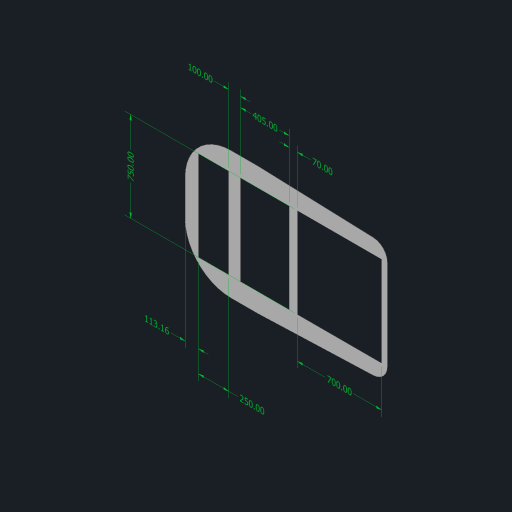
# Autodesk Inventor part: CHAPA_6
Saved by Autodesk Inventor 2024.3 (Build 283343000, 343)
## iProperties
Created: 2024-06-30
Part Number: CHAPA_6
Material: Generic
Document SubType Name: Sheet Metal
Designer: Niler
Density: 1 g/cm^3
Sheet Metal Rule: Default_mm
Appearance: Default
Author: Niler
Autodesk Inventor part; units mm, degrees
ref_plane "YZ Plane" through (0, 0, 0) normal (1, 0, 0) x (0, 1, 0)
ref_plane "XZ Plane" through (0, 0, 0) normal (0, 1, 0) x (-1, 0, 0)
ref_plane "XY Plane" through (0, 0, 0) normal (0, 0, 1) x (1, 0, 0)
sketch "Sketch1" plane through (0, 0, 0) normal (0, 0, 1) x (1, 0, 0)
  arc A0 (216.4448, 899.4448) -> (-166.5552, 516.4448) centre (216.4448, 516.4448) ccw
  line L0 (-166.5552, 216.4448) -> (-166.5552, 516.4448)
  arc A1 (-166.5552, 216.4448) -> (216.4448, -166.5552) centre (216.4448, 216.4448) ccw
  line L1 (443.4448, -166.5552) -> (216.4448, -166.5552)
  line L2 (216.4448, 899.4448) -> (443.4448, 899.4448)
  line L3 (443.5712, 899.4425) -> (1403.908, 864.732)
  line L4 (1403.908, -131.8425) -> (443.5712, -166.5529)
  arc A2 (443.4448, -166.5552) -> (443.5712, -166.5529) centre (443.4448, -163.0552) ccw
  arc A3 (443.5712, 899.4425) -> (443.4448, 899.4448) centre (443.4448, 895.9448) ccw
  arc A4 (1521.5977, 742.7757) -> (1403.908, 864.732) centre (1399.4977, 742.7117) ccw
  line L5 (1521.5977, 742.7757) -> (1521.6067, 725.4805)
  line L6 (1521.6067, 7.4091) -> (1521.5977, -9.8861)
  arc A5 (1403.908, -131.8425) -> (1521.5977, -9.8861) centre (1399.4977, -9.8222) ccw
  line L7 (1521.6067, 725.4805) -> (1521.6067, 7.4091)
  point P0 (0, 0)
extrude "Plate1" add sketch "Sketch1" along normal blind 1.5
sketch "Sketch2" plane through (0, 0, 1.5) normal (0, 0, 1) x (1, 0, 0)
  line L0 (771.6067, -8.5552) -> (1471.6067, -8.5552)
  line L1 (1471.6067, -8.5552) -> (1471.6067, 741.4448)
  line L2 (1471.6067, 741.4448) -> (771.6067, 741.4448)
  line L3 (771.6067, 741.4448) -> (771.6067, -8.5552)
  arc A0 (443.5712, 899.4425) -> (443.4448, 899.4448) centre (443.4448, 895.9448) ccw projected
  line L4 (216.4448, 899.4448) -> (443.4448, 899.4448) projected
  arc A1 (216.4448, 899.4448) -> (-166.5552, 516.4448) centre (216.4448, 516.4448) ccw projected
  line L5 (-166.5552, 216.4448) -> (-166.5552, 516.4448) projected
  arc A2 (-166.5552, 216.4448) -> (216.4448, -166.5552) centre (216.4448, 216.4448) ccw projected
  line L6 (443.4448, -166.5552) -> (216.4448, -166.5552) projected
  arc A3 (443.4448, -166.5552) -> (443.5712, -166.5529) centre (443.4448, -163.0552) ccw projected
  line L7 (1403.908, -131.8425) -> (443.5712, -166.5529) projected
  arc A4 (1403.908, -131.8425) -> (1521.5977, -9.8861) centre (1399.4977, -9.8222) ccw projected
  line L8 (1521.6067, 7.4091) -> (1521.5977, -9.8861) projected
  line L9 (1521.6067, 725.4805) -> (1521.6067, 7.4091) projected
  line L10 (1521.5977, 742.7757) -> (1521.6067, 725.4805) projected
  arc A5 (1521.5977, 742.7757) -> (1403.908, 864.732) centre (1399.4977, 742.7117) ccw projected
  line L11 (443.5712, 899.4425) -> (1403.908, 864.732) projected
  line L12 (296.6067, -8.5552) -> (701.6067, -8.5552)
  line L13 (701.6067, -8.5552) -> (701.6067, 741.4448)
  line L14 (701.6067, 741.4448) -> (296.6067, 741.4448)
  line L15 (296.6067, 741.4448) -> (296.6067, -8.5552)
  line L16 (-53.3933, -8.5552) -> (196.6067, -8.5552)
  line L17 (196.6067, -8.5552) -> (196.6067, 741.4448)
  line L18 (196.6067, 741.4448) -> (-53.3933, 741.4448)
  line L19 (-53.3933, 741.4448) -> (-53.3933, -8.5552)
  point P0 (0, 0)
  point P1 (1471.6067, 366.4448)
  point P2 (1521.6067, 366.4448)
  point P3 (701.6067, 366.4448)
  point P4 (771.6067, 366.4448)
  point P5 (196.6067, 366.4448)
  point P6 (296.6067, 366.4448)
  dimension "d1" = 50
  dimension "d2" = 750
  dimension "d3" = 700
  dimension "d4" = 750
  dimension "d5" = 70
  dimension "d6" = 405
  dimension "d7" = 750
  dimension "d8" = 100
  dimension "d9" = 250
  constraints: 24 end point, 6 midpoint, 6 parallel, 3 horizontal, 3 horizontal alignment, 3 perpendicular
  measures "d1" distance between parallel lines of L9 L1
  measures "d2" distance of L2.end L0.start
  measures "d3" distance of L0.start L0.end
  measures "d4" distance of L14.end L12.start
  measures "d5" distance between parallel lines of L3 L13
  measures "d6" distance of L13.end L14.end
  measures "d7" distance of L16.end L17.end
  measures "d8" distance between parallel lines of L15 L17
  measures "d9" distance of L17.end L18.end
extrude "Extrusion1" cut sketch "Sketch2" against normal through all contours L3 L2 L1 L0 | L15 L14 L13 L12 | L19 L18 L17 L16
equation "\"d0\" = Thickness"
equation "\"BendRadius\" = Thickness"
equation "\"BendReliefWidth\" = Thickness"
equation "\"BendReliefDepth\" = 0.5 * Thickness"
equation "\"CornerReliefSize\" = 4 * Thickness"
equation "\"MinimumRemnant\" = 2 * Thickness"
equation "\"TransitionRadius\" = BendRadius"
equation "\"JacobiRadiusSize\" = BendRadius"
equation "\"GapSize\" = Thickness"
equation "\"Thickness\" = 1.5"
body "Solid1"
